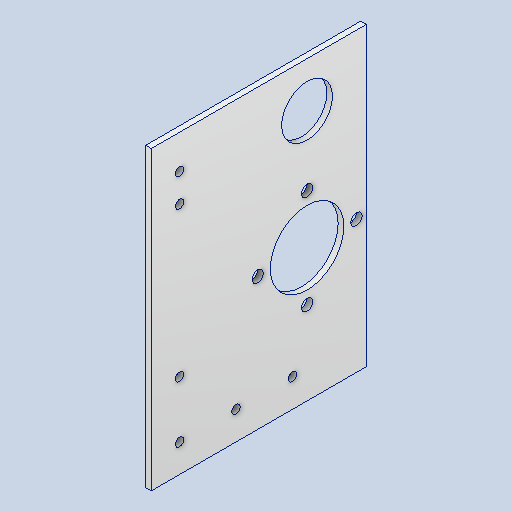
# Autodesk Inventor part: dribl-v1-Plate-3
Saved by Autodesk Inventor 2025.2 (Build 292293000, 293)
## iProperties
Created: 2025-01-07
Part Number: dribl-v1-Plate-3
Material: アルミニウム 6061
Document SubType Name: Modeling
Designer: haruy
Density: 2.7 g/cm^3
Appearance: アルミニウム - フラット
Author: haruy
Autodesk Inventor part; units mm, degrees
ref_plane "YZ Plane" through (0, 0, 0) normal (1, 0, 0) x (0, 1, 0)
ref_plane "XZ Plane" through (0, 0, 0) normal (0, 1, 0) x (-1, 0, 0)
ref_plane "XY Plane" through (0, 0, 0) normal (0, 0, 1) x (1, 0, 0)
derived "dribl-v1-ASP-Base.ipt"
sketch "スケッチ3" plane through (420, -432.3334, -303) normal (1, 0, 0) x (0, 0, -1)
  line L0 (20, 0) -> (20, 1308)
  line L1 (20, 102) -> (425, 102)
  line L2 (425, 102) -> (425, 122)
  line L3 (425, 122) -> (20, 122)
  line L4 (20, 122) -> (20, 102)
  circle A0 centre (55.18, 149) radius 21
  circle A1 centre (55.18, 191) radius 16
  circle A2 centre (55.18, 191) radius 13.68
  line L5 (0, 0) -> (20, 0)
  line L6 (0, 0) -> (20, 0)
  line L7 (0, 0) -> (484, 0)
  line L8 (484, 0) -> (484, -20)
  line L9 (484, -20) -> (0, -20)
  line L10 (0, -20) -> (0, 0)
  line L11 (75.18, 1308) -> (94.3557, 1313.6826)
  line L12 (94.3557, 1313.6826) -> (480.203, 11.6512)
  line L13 (480.203, 11.6512) -> (461.0273, 5.9686)
  line L14 (461.0273, 5.9686) -> (75.18, 1308)
  line L15 (0, 1308) -> (0, 0)
  line L16 (0, 207) -> (55.18, 207)
  line L17 (76.18, 149) -> (76.18, 102)
  line L18 (76.18, 149) -> (76.18, 207)
  line L19 (76.18, 207) -> (55.18, 207)
  circle A3 centre (10, 195) radius 1.5
  circle A4 centre (10, 185) radius 1.5
  line L20 (55.18, 175) -> (0, 175)
  circle A5 centre (30, 112) radius 1.5
  circle A6 centre (50, 112) radius 1.5
  line L21 (20, 102) -> (0, 102)
  circle A7 centre (10, 112) radius 1.5
  circle A8 centre (10, 132) radius 1.5
  circle A9 centre (55.18, 1292) radius 16
  line L22 (20, 1308) -> (0, 1308)
  line L23 (0, 1308) -> (55.18, 1308)
  line L24 (55.18, 1276) -> (0, 1276)
  line L25 (55.18, 1308) -> (75.18, 1308)
  circle A10 centre (55.18, 191) radius 9
  circle A11 centre (55.18, 149) radius 13
  circle A12 centre (55.18, 149) radius 17.5
  circle A13 centre (55.18, 166.5) radius 2
  circle A14 centre (37.68, 149) radius 2
  circle A15 centre (55.18, 131.5) radius 2
  circle A16 centre (72.68, 149) radius 2
  circle A17 centre (55.18, 1292) radius 7.5
  line L26 (55.18, 1276) -> (84.663, 1276)
  circle A18 centre (10, 1296) radius 1.5
  circle A19 centre (10, 1286) radius 1.5
  circle A20 centre (87.6092, 1301.2534) radius 1.5
  circle A21 centre (90.4504, 1291.6656) radius 1.5
  line L27 (84.663, 1276) -> (103.8387, 1281.6826)
  point P0 (-303, 432.3334)
  dimension "d3" = 35
  dimension "d1" = 18
  dimension "d2" = 26
  dimension "d4" = 4
  dimension "d5" = 0
  dimension "d8" = 360
  measures "d1" diameter of A10
  measures "d2" diameter of A11
  measures "d4" diameter of A13
  measures "d5" horizontal distance of point (55.18, 149) A13.centre
sketch "スケッチ4" plane through (400, -241.3334, -323) normal (0, -1, 0) x (1, 0, 0)
  line L0 (20, 20) -> (20, 0)
  line L1 (20, 20) -> (20, -84.1399)
  line L2 (20, 20) -> (-44.5955, 20)
  line L3 (20, -35.18) -> (-46.4938, -35.18)
  line L4 (0, 0) -> (20, 0)
  line L5 (-35, 20) -> (-35, -35.18)
  line L6 (-35, -35.18) -> (-5, -35.18)
  line L7 (-5, -35.18) -> (-5, -5.18)
  line L8 (-5, -5.18) -> (-35, -5.18)
  line L9 (-35, -5.18) -> (-35, -35.18)
  line L10 (0, 0) -> (0, 20)
  line L11 (16.5, -21.5) -> (3.5, -21.5)
  line L12 (3.5, -21.5) -> (3.5, -48.86)
  line L13 (3.5, -48.86) -> (16.5, -48.86)
  line L14 (16.5, -48.86) -> (16.5, -21.5)
  line L15 (-590, 20) -> (-610, 20)
  line L16 (-590, 20) -> (0, 20)
  line L17 (-295, 20) -> (-295, -284.0513)
  line L18 (-555, 20) -> (-555, -35.18)
  line L19 (-585, -5.18) -> (-555, -5.18)
  line L20 (-555, -35.18) -> (-585, -35.18)
  line L21 (-610, -35.18) -> (-543.5062, -35.18)
  line L22 (-585, -35.18) -> (-585, -5.18)
  line L23 (-606.5, -21.5) -> (-593.5, -21.5)
  line L24 (-593.5, -21.5) -> (-593.5, -48.86)
  line L25 (-593.5, -48.86) -> (-606.5, -48.86)
  line L26 (-606.5, -48.86) -> (-606.5, -21.5)
  point P0 (-400, 323)
ref_plane "作業平面1" through (105, -432.3334, -303) normal (-1, 0, 0) x (0, 0, 1)
ref_plane "作業平面2" through (400, -241.3334, -323) normal (0, -1, 0) x (1, 0, 0)
extrude "押し出し1" add sketch "スケッチ3" against normal blind 2 contours L21 L15 L20 L0 | L0 L3 L17 L1 | A0 | L0 L20 A1 L19 L18 L17 L3 | L20 L15 L16 L0 | L0 L16 A1 L20 | A1 | A2 | A16 A12 A15 A14 A13
sketch "スケッチ2" plane through (400, -432.3334, -303) normal (0, 0, 1) x (1, 0, 0)
  line L0 (-590, 1308) -> (-590, 0) projected
  line L1 (-590, 150) -> (0, 150) projected
  line L2 (0, 150) -> (0, 170) projected
  line L3 (0, 170) -> (-590, 170) projected
  line L4 (-590, 170) -> (-590, 150) projected
  line L5 (0, 0) -> (20, 0) projected
  circle A0 centre (-35, 191) radius 13.68 construction
  line L6 (0, 1308) -> (0, 0) projected
  circle A1 centre (-35, 191) radius 16 projected
  line L7 (-295, 150) -> (-295, 0) projected
  circle A2 centre (-555, 191) radius 16 projected
  circle A3 centre (-555, 191) radius 13.68 construction
  circle A4 centre (-35, 191) radius 9 projected
  line L8 (-3, 170) -> (-21.4335, 199.4823) projected
  line L9 (-51, 191) -> (-51, 150) projected
  circle A5 centre (-30, 160) radius 1.5 projected
  circle A6 centre (-10, 160) radius 1.5 projected
  circle A7 centre (10, 160) radius 1.5 projected
  circle A8 centre (10, 140) radius 1.5 projected
  line L10 (0, 170) -> (20, 170) projected
  line L11 (0, 130) -> (20, 130) projected
  line L12 (20, 1308) -> (20, 0) projected
  line L13 (20, 170) -> (20, 130) projected
  line L14 (0, 130) -> (0, 150) projected
  circle A9 centre (-600, 140) radius 1.5 projected
  line L15 (-590, 130) -> (-610, 130) projected
  circle A10 centre (-600, 160) radius 1.5 projected
  line L16 (-590, 170) -> (-610, 170) projected
  circle A11 centre (-580, 160) radius 1.5 projected
  circle A12 centre (-560, 160) radius 1.5 projected
  line L17 (-539, 191) -> (-539, 150) projected
  line L18 (-587, 170) -> (-568.5665, 199.4823) projected
  circle A13 centre (-555, 191) radius 9 projected
  line L19 (-590, 130) -> (-590, 170) projected
  line L20 (-610, 170) -> (-610, 130) projected
  line L21 (-609, 1308) -> (-609, 0) projected
  point P0 (-400, 432.3334)
